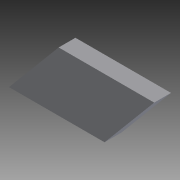
# Autodesk Inventor part: Bad hopper design_v1
Saved by Autodesk Inventor 2013 (Build 170138000, 138)
## iProperties
Created: 2013-01-14
Part Number: Bad hopper design_v1
Material: Generic
Document SubType Name: Modeling
Designer: motoennies
Density: 1 g/cm^3
Author: motoennies
Autodesk Inventor part; units mm, degrees
ref_plane "YZ Plane" through (0, 0, 0) normal (1, 0, 0) x (0, 1, 0)
ref_plane "XZ Plane" through (0, 0, 0) normal (0, 1, 0) x (-1, 0, 0)
ref_plane "XY Plane" through (0, 0, 0) normal (0, 0, 1) x (1, 0, 0)
sketch "Sketch1" plane through (0, 0, 0) normal (0, 0, 1) x (1, 0, 0)
  line L0 (0, 0) -> (288.925, 0)
  line L1 (0, 0) -> (150.076, 178.8536)
  line L2 (288.925, 0) -> (439.001, 178.8536)
  line L3 (150.076, 178.8536) -> (439.001, 178.8536)
  line L4 (150.076, 178.8536) -> (294.5385, 178.8536) construction
  line L5 (294.5385, 178.8536) -> (144.4625, 0) construction
  dimension "d0" = 288.925
  dimension "d1" = 233.4768
  dimension "d2" = 50
  dimension "d3" = 233.4768
  dimension "d4" = 144.4625
  constraints: 12 end point, 2 midpoint, 2 parallel, 1 horizontal
  measures "d0" distance of L0.start L0.end
  measures "d1" distance of L0.start L1.end
  measures "d2" angle of L0 L1
  measures "d3" distance of L0.end L2.end
  measures "d4" distance of L1.end L4.end
extrude "Extrusion1" add sketch "Sketch1" along normal blind 50.8
body "Solid1"
